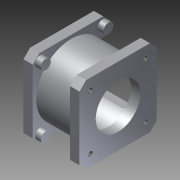
# Autodesk Inventor part: GL20NU1 Y Motor bracket
Saved by Autodesk Inventor 2011 SP1 (Build 150282100, 282)
## iProperties
Created: 2013-11-12
Part Number: GL20NU1 Y Motor bracket
Catalog Web Link: www.cadenas.de
Description: Type GL-N-Y-Motor bracket-
Vendor: THK
Document SubType Name: Modeling
Designer: PARTuser1
Manufacturer: THK
Density: 1 g/cm^3
Category: PARTsolutions
Company: THK
Title: GL20NU1 Y Motor bracket
Author: Cadenas PARTsolutions
PSOL_IDENT_0: {$CADENAS_DATA\23d-libs\thk\actuator\type_gl_n\type_gl_n_f_na_ex.prj},212 {VTYP=3D},{NB=GL20NU1 Y Mo
PSOL_IDENT_1: tor bracket},{LINA=GL20NU1 Y Motor bracket},{NN=Type GL-N-Y-Motor bracket},{DATE=01.03.2011 00:58:01
PSOL_IDENT_2: },{GEOMDATE=25.01.2011 00:19:00},{VERSION=},{LINEID=20},{LINESUBID=-1},{WBVAR=TB,R1}  {NB=GL20NU1 Y
PSOL_IDENT_3: Motor bracket},{LINA=GL20NU1 Y Motor bracket},{KT=DUMMY},{IDNR=},{MN=GL20N},{TB=U1},{D=19.075},{D1=2
PSOL_IDENT_4: 5},{NDM=2},{L1=66},{VER=1},{PCD=47.14},{B=8},{L2=32},{H=77.98},{LX=50.5},{L3=60},{R=14},{R1=},{NDM1=
PSOL_IDENT_5: 2},{P=10},{A=25},{B1=29},{DS=Ex},{RX='','None'},{TB1='B1', 'B1 : inner diameter  50, dia. 5.5, PCD60
PSOL_IDENT_6: ', 'B2'  , 'B2 : inner diameter  60, dia. 6.5, PCD90', 'U1'  , 'U1 : inner diameter  38.1, M4, PCD80
PSOL_IDENT_7: ', 'V1'  , 'V1:inner diameter 73.03,M5'},{BT=38},{BW=35},{BD=8},{BOD=30}
CNS_NN: Type GL-N-Y-Motor bracket
CNS_NB: GL20NU1 Y Motor bracket
CNS_NBSYN: $MN.$TB.$R1. Y Motor bracket
CNS_LINA: GL20NU1 Y Motor bracket
CNS_MN: GL20N
CNS_TB: U1 : inner diameter  38.1, M4, PCD80
CNS_D: 19.075
CNS_D1: 25.000
CNS_NDM: 2.000
CNS_L1: 66.000
CNS_VER: 1
CNS_PCD: 47.140
CNS_B: 8.000
CNS_L2: 32.000
CNS_H: 77.980
CNS_LX: 50.500
CNS_L3: 60.000
CNS_R: 14.000
CNS_NDM1: 2.000
CNS_P: 10.000
CNS_A: 25.000
CNS_B1: 29.000
CNS_DS: Ex
CNS_RX: '','None'
CNS_TB1: 'B1', 'B1 : inner diameter  50, dia. 5.5, PCD60', 'B2'  , 'B2 : inner diameter  60, dia. 6.5, PCD90', 'U1'  , 'U1 : inner diameter  38.1, M4, PCD80', 'V1'  , 'V1:inner diameter 73.03,M5'
CNS_BT: 38.000
CNS_BW: 35.000
CNS_BD: 8.000
CNS_BOD: 30.000
SUPPLIER: THK
ARTICLENO: GL20NU1 Y Motor bracket
BOMINFO: GL20NU1 Y Motor bracket
CREATOR: CADENAS GmbH
Autodesk Inventor part; units mm, degrees
sketch "Sketch_1" plane through (0, 0, 0) normal (1, 0, 0) x (0, 1, 0)
  line L0 (27.33, 32.99) -> (-27.33, 32.99)
  line L1 (-27.33, 32.99) -> (-32.99, 27.33)
  line L2 (-32.99, 27.33) -> (-32.99, -27.33)
  line L3 (-32.99, -27.33) -> (-27.33, -32.99)
  line L4 (-27.33, -32.99) -> (27.33, -32.99)
  line L5 (27.33, -32.99) -> (32.99, -27.33)
  line L6 (32.99, -27.33) -> (32.99, 27.33)
  line L7 (32.99, 27.33) -> (27.33, 32.99)
  constraints: 16 end point
extrude "Extrusion1" add sketch "Sketch_1" along normal blind 8
sketch "Sketch_2" plane through (0, 0, 0) normal (0, 0, 1) x (1, 0, 0)
  line L0 (40, 0) -> (8, 0)
  line L1 (8, 0) -> (8, 30)
  line L2 (8, 30) -> (40, 30)
  line L3 (40, 30) -> (40, 0)
  line L4 (40, 0) -> (8, 0)
  constraints: 10 end point
revolve "Revolution1" add sketch "Sketch_2" angle 360 about axis through (40, 0, 0) along (1, 0, 0)
sketch "Sketch_3" plane through (40, 0, 0) normal (1, 0, 0) x (0, 0, -1)
  line L0 (-33, 27.34) -> (-33, -27.34)
  line L1 (-33, -27.34) -> (-27.34, -33)
  line L2 (-27.34, -33) -> (27.34, -33)
  line L3 (27.34, -33) -> (33, -27.34)
  line L4 (33, -27.34) -> (33, 27.34)
  line L5 (33, 27.34) -> (27.34, 33)
  line L6 (27.34, 33) -> (-27.34, 33)
  line L7 (-27.34, 33) -> (-33, 27.34)
  constraints: 16 end point
extrude "Extrusion2" add sketch "Sketch_3" along normal blind 8
sketch "Sketch4" plane through (48, 0, 0) normal (1, 0, 0) x (0, 0, -1)
  point P0 (0, 0)
hole "Drilling 1" at (48, 0, 0) direction (-1, 0, 0) diameter 38.15 depth 8
sketch "Sketch5" plane through (40, 0, 0) normal (1, 0, 0) x (0, 0, -1)
  point P0 (0, 0)
hole "Drilling 2" at (40, 0, 0) direction (-1, 0, 0) diameter 50 depth 40
sketch "Sketch_7" plane through (0, 26.87, 0) normal (0, 1, 0) x (1, 0, 0)
  line L0 (13, 26.87) -> (8, 26.87)
  line L1 (8, 26.87) -> (8, 31.12)
  line L2 (8, 31.12) -> (13, 31.12)
  line L3 (13, 31.12) -> (13, 26.87)
  line L4 (13, 26.87) -> (8, 26.87)
  constraints: 10 end point
revolve "Revolution2" add sketch "Sketch_7" angle 360 about axis through (13, 26.87, -26.87) along (1, 0, 0)
sketch "Sketch_8" plane through (0, 26.87, 0) normal (0, 1, 0) x (1, 0, 0)
  line L0 (13, -26.87) -> (8, -26.87)
  line L1 (8, -26.87) -> (8, -22.62)
  line L2 (8, -22.62) -> (13, -22.62)
  line L3 (13, -22.62) -> (13, -26.87)
  line L4 (13, -26.87) -> (8, -26.87)
  constraints: 10 end point
revolve "Revolution3" add sketch "Sketch_8" angle 360 about axis through (13, 26.87, 26.87) along (1, 0, 0)
sketch "Sketch8" plane through (48, 0, 0) normal (1, 0, 0) x (0, 0, -1)
  point P0 (-23.57, 23.57)
hole "Drilling 3" at (48, 23.57, 23.57) direction (-1, 0, 0) diameter 3.242 depth 8 countersink diameter 4 countersink angle 90 thread size "M4x0.7" class "6H" standard "ISO Metric profile"
sketch "Sketch9" plane through (48, 0, 0) normal (1, 0, 0) x (0, 0, -1)
  point P0 (-23.57, -23.57)
hole "Drilling 4" at (48, -23.57, 23.57) direction (-1, 0, 0) diameter 3.242 depth 8 countersink diameter 4 countersink angle 90 thread size "M4x0.7" class "6H" standard "ISO Metric profile"
sketch "Sketch10" plane through (48, 0, 0) normal (1, 0, 0) x (0, 0, -1)
  point P0 (23.57, 23.57)
hole "Drilling 5" at (48, 23.57, -23.57) direction (-1, 0, 0) diameter 3.242 depth 8 countersink diameter 4 countersink angle 90 thread size "M4x0.7" class "6H" standard "ISO Metric profile"
sketch "Sketch11" plane through (48, 0, 0) normal (1, 0, 0) x (0, 0, -1)
  point P0 (23.57, -23.57)
hole "Drilling 6" at (48, -23.57, -23.57) direction (-1, 0, 0) diameter 3.242 depth 8 countersink diameter 4 countersink angle 90 thread size "M4x0.7" class "6H" standard "ISO Metric profile"
sketch "Sketch_9" plane through (0, -26.87, 0) normal (0, 1, 0) x (1, 0, 0)
  line L0 (13, 26.87) -> (8, 26.87)
  line L1 (8, 26.87) -> (8, 31.12)
  line L2 (8, 31.12) -> (13, 31.12)
  line L3 (13, 31.12) -> (13, 26.87)
  line L4 (13, 26.87) -> (8, 26.87)
  constraints: 10 end point
revolve "Revolution4" add sketch "Sketch_9" angle 360 about axis through (13, -26.87, -26.87) along (1, 0, 0)
sketch "Sketch_10" plane through (0, -26.87, 0) normal (0, 1, 0) x (1, 0, 0)
  line L0 (13, -26.87) -> (8, -26.87)
  line L1 (8, -26.87) -> (8, -22.62)
  line L2 (8, -22.62) -> (13, -22.62)
  line L3 (13, -22.62) -> (13, -26.87)
  line L4 (13, -26.87) -> (8, -26.87)
  constraints: 10 end point
revolve "Revolution5" add sketch "Sketch_10" angle 360 about axis through (13, -26.87, 26.87) along (1, 0, 0)
sketch "Sketch_33" plane through (0, 0, 0) normal (0, 1, 0) x (-1, 0, 0)
  line L0 (0, -17.5) -> (0, 17.5)
  line L1 (0, 17.5) -> (-33, 17.5)
  arc A0 (-33, 17.5) -> (-38, 12.5) centre (-33, 12.5) ccw
  line L2 (-38, 12.5) -> (-38, -12.5)
  arc A1 (-38, -12.5) -> (-33, -17.5) centre (-33, -12.5) ccw
  line L3 (-33, -17.5) -> (0, -17.5)
  constraints: 8 end point, 4 point on circle, 2 centre point
extrude "Extrusion3" cut sketch "Sketch_33" along normal blind 33
ref_plane "type_gl_n_bm_XY" through (0, 0, 0) normal (1, 0, 0) x (0, -1, 0)
ref_plane "type_gl_n_bm_YZ" through (0, 0, 0) normal (0, -1, 0) x (0, 0, -1)
ref_plane "type_gl_n_bm_ZX" through (0, 0, 0) normal (0, 0, -1) x (1, 0, 0)
body "Solid1"
